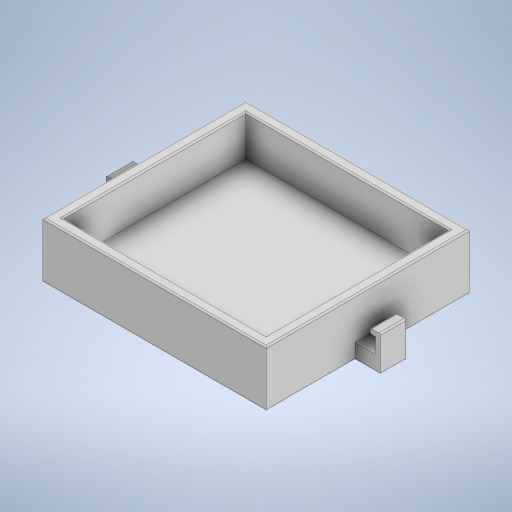
# Autodesk Inventor part: obudowa
Saved by Autodesk Inventor 2024.2 (Build 282272000, 272)
## iProperties
Created: 2024-05-03
Part Number: obudowa
Material: Ogólny
Document SubType Name: Modeling
Designer: kacpe
Density: 1 g/cm^3
Appearance: Domyślna
Author: kacpe
Autodesk Inventor part; units mm, degrees
ref_plane "YZ Plane" through (0, 0, 0) normal (1, 0, 0) x (0, 1, 0)
ref_plane "XZ Plane" through (0, 0, 0) normal (0, 1, 0) x (-1, 0, 0)
ref_plane "XY Plane" through (0, 0, 0) normal (0, 0, 1) x (1, 0, 0)
sketch "Szkic1" plane through (0, 0, 0) normal (0, 1, 0) x (-1, 0, 0)
  line L0 (0, 0) -> (0, -40)
  line L1 (0, 0) -> (44, 0)
  line L2 (44, 0) -> (44, -40)
  line L3 (0, -40) -> (44, -40)
  dimension "d0" = 40
  dimension "d1" = 44
  constraints: 8 end point, 2 vertical, 1 horizontal, 1 perpendicular
  measures "d0" distance of L0.start L0.end
  measures "d1" distance of L0.start L1.end
extrude "Wyciągnięcie proste1" add sketch "Szkic1" along normal blind 3
sketch "Szkic2" plane through (0, 3, 0) normal (0, 1, 0) x (1, 0, 0)
  line L0 (0, 0) -> (0, 40) projected
  line L1 (0, 40) -> (-44, 40) projected
  line L2 (-44, 40) -> (-44, 0) projected
  line L3 (-44, 0) -> (0, 0) projected
  line L4 (-42, 2) -> (-42, 38)
  line L5 (-42, 38) -> (-2, 38)
  line L6 (-2, 38) -> (-2, 2)
  line L7 (-2, 2) -> (-42, 2)
  dimension "d4" = 2
  constraints: 8 end point, 3 other
  measures "d4" distance between parallel lines of L2 L4
extrude "Wyciągnięcie proste2" add sketch "Szkic2" along normal blind 8
sketch "Szkic3" plane through (0, 0, 0) normal (0, -1, 0) x (1, 0, 0)
  line L0 (0, 0) -> (0, -40) projected
  line L1 (-44, 0) -> (0, 0) projected
  line L2 (-44, -40) -> (-44, 0) projected
  line L3 (0, -40) -> (-44, -40) projected
  line L4 (0, -20) -> (5, -20)
  line L5 (-44, -20) -> (-49, -20) construction
  line L6 (-49, -20) -> (-49, -22.5)
  line L7 (-49, -20) -> (-49, -17.5)
  line L8 (5, -20) -> (5, -22.5)
  line L9 (5, -22.5) -> (5, -20)
  line L10 (5, -20) -> (5, -17.5)
  line L11 (5, -17.5) -> (0, -17.5)
  line L12 (5, -22.5) -> (0, -22.5)
  line L13 (-49, -22.5) -> (-44, -22.5)
  line L14 (-49, -17.5) -> (-44, -17.5)
  dimension "d7" = 5
  dimension "d8" = 5
  dimension "d9" = 2.5
  dimension "d10" = 2.5
  dimension "d11" = 2.5
  dimension "d12" = 2.5
  constraints: 22 end point, 6 point on line, 3 perpendicular, 2 equal length, 2 horizontal, 2 midpoint, 2 vertical
  measures "d7" distance of L4.start L4.end
  measures "d8" distance of L5.start L5.end
  measures "d9" distance of L5.end L6.end
  measures "d10" distance of L5.end L7.end
  measures "d11" distance of L4.end L8.end
  measures "d12" distance of L4.end L10.end
extrude "Wyciągnięcie proste3" add sketch "Szkic3" against normal blind 3 contours L11 L10 L4 L0 | L4 L8 L12 L0 | L2 L13 L6 L7 L14
sketch "Szkic4" plane through (0, 3, 0) normal (0, 1, 0) x (1, 0, 0)
  line L0 (5, 17.5) -> (5, 22.5) projected
  line L1 (5, 22.5) -> (0, 22.5) projected
  line L2 (0, 17.5) -> (0, 22.5) projected
  line L3 (0, 17.5) -> (5, 17.5) projected
  line L4 (5, 17.5) -> (4, 17.5)
  line L5 (4, 17.5) -> (4, 22.5)
  line L6 (4, 22.5) -> (5, 22.5)
  line L7 (5, 22.5) -> (5, 17.5)
  line L8 (-49, 22.5) -> (-49, 17.5) projected
  line L9 (-49, 17.5) -> (-44, 17.5) projected
  line L10 (-44, 22.5) -> (-44, 17.5) projected
  line L11 (-44, 22.5) -> (-49, 22.5) projected
  line L12 (-49, 17.5) -> (-48, 17.5)
  line L13 (-48, 17.5) -> (-48, 22.5)
  line L14 (-48, 22.5) -> (-49, 22.5)
  line L15 (-49, 22.5) -> (-49, 17.5)
  point P0 (0, 0)
  dimension "d15" = 1
  dimension "d16" = 1
  constraints: 16 end point, 4 parallel, 2 horizontal, 2 perpendicular, 2 point on line
  measures "d15" distance of L5.end L6.end
  measures "d16" distance of L14.end L13.end
extrude "Wyciągnięcie proste4" add sketch "Szkic4" along normal blind 4 contours L3 L5 L1 L0 | L11 L13 L9 L8
sketch "Szkic5" plane through (4, 3, -22.5) normal (-1, 0, 0) x (0, 0, 1)
  line L0 (5, 0) -> (0, 0) projected
  line L1 (5, 0) -> (5, 4) projected
  line L2 (0, 4) -> (5, 4) projected
  line L3 (0, 0) -> (0, 4) projected
  line L4 (5, 4) -> (0, 4)
  line L5 (0, 4) -> (0, 3)
  line L6 (0, 3) -> (5, 3)
  line L7 (5, 3) -> (5, 4)
  point P0 (22.5, -3)
  dimension "d19" = 5
  dimension "d20" = 1
  constraints: 8 end point, 2 parallel, 1 horizontal, 1 perpendicular
  measures "d19" distance of L6.end L5.end
  measures "d20" distance of L5.end L4.end
extrude "Wyciągnięcie proste5" add sketch "Szkic5" along normal blind 1 contours L6 L3 L2 L1
sketch "Szkic6" plane through (-48, 3, -17.5) normal (1, 0, 0) x (0, 0, -1)
  line L0 (5, 0) -> (0, 0) projected
  line L1 (5, 0) -> (5, 4) projected
  line L2 (0, 4) -> (5, 4) projected
  line L3 (0, 0) -> (0, 4) projected
  line L4 (0, 4) -> (5, 4)
  line L5 (5, 4) -> (5, 3)
  line L6 (5, 3) -> (0, 3)
  line L7 (0, 3) -> (0, 4)
  point P0 (-17.5, -3)
  point P1 (0, 3)
  point P2 (5, 3)
  dimension "d23" = 5
  dimension "d24" = 1
  constraints: 8 end point, 2 parallel, 1 horizontal, 1 perpendicular
  measures "d23" distance of L5.end L6.end
  measures "d24" distance of L4.end L5.end
extrude "Wyciągnięcie proste6" add sketch "Szkic6" along normal blind 1 contours L6 L3 L2 L1
fillet "Zaokrąglenie1" radius 0.3 26 edges at (-49, 0, -20) (5, 0, -20) (5, 7, -20) (-49, 7, -20) (-22, 0, -40) (-44, 0, -31.25) (0, 0, -31.25) (0, 0, -8.75) (2.5, 0, -17.5) (2.5, 0, -22.5) (-22, 0, 0) (-44, 0, -8.75) (-46.5, 0, -17.5) (-46.5, 0, -22.5) (-2, 11, -20) (0, 11, -20) (-22, 11, -2) (-22, 11, 0) (-22, 11, -38) (-22, 11, -40) (-42, 11, -20) (-44, 11, -20) (-47, 7, -20) (3, 7, -20) (3, 6, -20) (-47, 6, -20)
